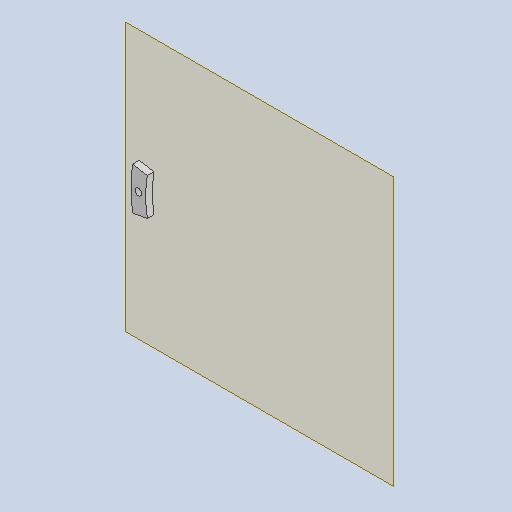
# Autodesk Inventor part: Montage_Ring_Vorne_Aufdickung_Gewinde
Saved by Autodesk Inventor 2022.2 (Build 262287010, 287A)
## iProperties
Created: 2024-01-10
Part Number: Montage_Ring_Vorne_Aufdickung_Gewinde
Material: Generisch
Document SubType Name: Modeling
Designer: ppovolni
Density: 1 g/cm^3
Appearance: Vorgabe
Author: ppovolni
Autodesk Inventor part; units mm, degrees
ref_plane "YZ Plane" through (0, 0, 0) normal (1, 0, 0) x (0, 1, 0)
ref_plane "XZ Plane" through (0, 0, 0) normal (0, 1, 0) x (-1, 0, 0)
ref_plane "XY Plane" through (0, 0, 0) normal (0, 0, 1) x (1, 0, 0)
ref_plane "Arbeitsebene1" through (0, 0, 0) normal (0, 0, 1) x (1, 0, 0)
sketch "Skizze1" plane through (0, 0, 0) normal (0, 0, 1) x (1, 0, 0)
  circle A0 centre (86.2, 0) radius 2.6 construction
  circle A1 centre (-86.2, 0) radius 2.6 construction
  circle A2 centre (0, 0) radius 91.8 construction
  arc A3 (5.5, 85.9242) -> (-5.5, 85.9242) centre (0, 0) ccw construction
  line L0 (5.5, 85.9242) -> (5.5, 80.4121) construction
  arc A4 (-5.5, 80.4121) -> (5.5, 80.4121) centre (0, 0) ccw construction
  line L1 (-5.5, 80.4121) -> (-5.5, 85.9242) construction
  arc A5 (-90.4054, 15.9409) -> (-90.4054, -15.9409) centre (0, 0) ccw
  arc A6 (-79.3755, 13.996) -> (-79.3755, -13.996) centre (0, 0) ccw
  line L2 (-90.4054, 15.9409) -> (0, 0) construction
  line L3 (0, 0) -> (-90.4054, -15.9409) construction
  line L4 (-90.4054, 15.9409) -> (-79.3755, 13.996)
  line L5 (-79.3755, -13.996) -> (-90.4054, -15.9409)
  line L6 (0, 0) -> (-86.2, 0) construction
  circle A7 centre (-86.2, 0) radius 2.6
  dimension "d0" = 10
  dimension "d1" = 10
  constraints: 10 end point, 6 point on circle, 3 centre point, 3 coincident, 2 collinear, 2 concentric, 2 point on line, 1 horizontal, 2 other
  measures "d0" angle of L6 L2
  measures "d1" angle of L3 L6
extrude "Extrusion1" add sketch "Skizze1" along normal blind 5
